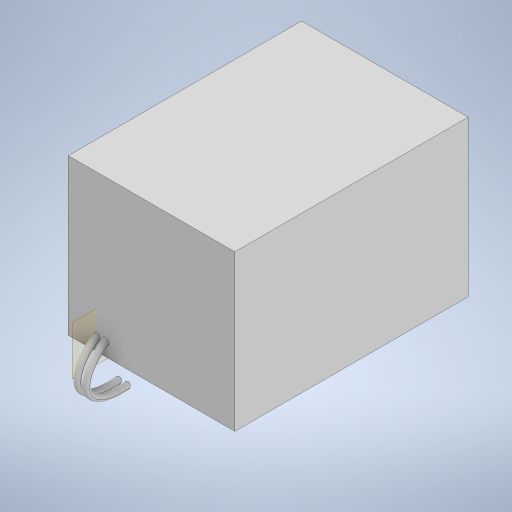
# Autodesk Inventor part: battery
Saved by Autodesk Inventor 2023 (Build 270158000, 158)
## iProperties
Created: 2023-03-23
Part Number: battery
Material: 一般
Document SubType Name: Modeling
Designer: 310611102
Density: 1 g/cm^3
Appearance: 預設
Author: 310611102
Autodesk Inventor part; units mm, degrees
ref_plane "YZ Plane" through (0, 0, 0) normal (1, 0, 0) x (0, 1, 0)
ref_plane "XZ Plane" through (0, 0, 0) normal (0, 1, 0) x (-1, 0, 0)
ref_plane "XY Plane" through (0, 0, 0) normal (0, 0, 1) x (1, 0, 0)
sketch "Sketch1" plane through (0, 0, 0) normal (0, 0, 1) x (1, 0, 0)
  line L0 (-37.5, 35) -> (37.5, 35)
  line L1 (37.5, 35) -> (37.5, -35)
  line L2 (37.5, -35) -> (-37.5, -35)
  line L3 (-37.5, -35) -> (-37.5, 35)
  line L4 (-37.5, 35) -> (37.5, -35) construction
  line L5 (37.5, 35) -> (-37.5, -35) construction
  point P0 (0, 0)
  dimension "d0" = 75
  dimension "d1" = 70
  constraints: 12 end point, 2 midpoint, 2 parallel, 1 horizontal, 1 perpendicular
  measures "d0" distance of L0.start L0.end
  measures "d1" distance of L2.end L0.start
extrude "Extrusion1" add sketch "Sketch1" along normal blind 105
sketch "Sketch2" plane through (0, 0, 105) normal (0, 0, 1) x (1, 0, 0)
  circle A0 centre (-24.7933, -29.2153) radius 1.5
  circle A1 centre (-20.7933, -29.2153) radius 1.5
  point P0 (0, 0)
  dimension "d4" = 3
  dimension "d5" = 3
  dimension "d6" = 4
  constraints: 2 centre point, 1 horizontal alignment
  measures "d4" diameter of A0
  measures "d5" diameter of A1
  measures "d6" distance of A1.centre A0.centre
ref_plane "Work Plane2" through (-24.7933, -29.2153, 105) normal (1, 0, 0) x (0, 1, 0)
sketch "Sketch3" plane through (-24.7933, -29.2153, 105) normal (1, 0, 0) x (0, 1, 0)
  line L0 (0, 0) -> (-8.28, 12.6748) construction
  line L1 (-8.28, 12.6748) -> (-23.4846, 12.6748) construction
  line L2 (-23.4846, 12.6748) -> (-21.9413, -9.551) construction
  spline S0 degree 3 poles (0, 0) (-8.28, 12.6748) (-23.4846, 12.6748) (-21.9413, -9.551) knots 1 1 1 1 2 2 2 2
  point P0 (29.2153, -105)
  constraints: 1 horizontal, 3 other
sweep "Sweep1" add profiles "Sketch2" path "Sketch3" contours A0
pattern_linear "Rectangular Pattern1" count 2 spacing 4 along (1, 0, 0) of "Sweep1"
body "Solid1"
